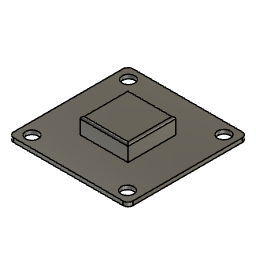
GYSFDMAXB (Autodesk Fusion 360 design; units mm, degrees)
Autodesk Fusion 360 part; units mm, degrees
sketch "スケッチ1" plane through (0, 0, 0) normal (0, 0, 1) x (1, 0, 0)
  line L0 (0, 0) -> (30, 0)
  line L1 (30, 0) -> (0, 0)
  line L2 (0, 0) -> (0, 30)
  line L3 (0, 30) -> (30, 30)
  line L4 (30, 30) -> (30, 0)
  line L5 (0, 0) -> (1.25, 0)
  line L6 (0, 0) -> (0, 1.25)
  arc A0 (0, 1.25) -> (1.25, 0) centre (1.25, 1.25) ccw
  arc A1 (1.25, 30) -> (0, 28.75) centre (1.25, 28.75) ccw
  arc A2 (30, 28.75) -> (28.75, 30) centre (28.75, 28.75) ccw
  arc A3 (28.75, 0) -> (30, 1.25) centre (28.75, 1.25) ccw
  line L7 (0, 30) -> (0, 28.73)
  circle A4 centre (3, 27.13) radius 1.6
  circle A5 centre (27, 27.13) radius 1.6
  circle A6 centre (27, 2.87) radius 1.6
  circle A7 centre (3, 2.87) radius 1.6
  dimension "d1" = 30
  dimension "d2" = 1.25
  dimension "d3" = 1.25
  dimension "d4" = 1.27
  dimension "d6" = 3.2
  constraint coincident L0.start L1.end
  constraint horizontal L0
  constraint horizontal L1
  constraint vertical L2
  constraint horizontal L3
  constraint vertical L4
  constraint perpendicular L2 L5
  constraint perpendicular L5 L6
  constraint perpendicular L3 L7
  measures "d1" distance of L0.start L0.end
  measures "d2" distance of L0.start L5.end
  measures "d3" distance of L0.start L6.end
  measures "d4" distance of L2.end L7.end
  measures "d6" diameter of A4
extrude "押し出し1" add sketch "スケッチ1" along normal blind 1 contours L0 L1 L2 L3 L4 A0 A1 A2 A3 L7
sketch "スケッチ2" plane through (0, 0, 1) normal (0, 0, 1) x (-1, 0, 0)
  circle A0 centre (-3, -27.13) radius 1.6
  circle A1 centre (-3, -2.87) radius 1.6
  circle A2 centre (-27, -2.87) radius 1.6
  circle A3 centre (-27, -27.13) radius 1.6
  arc A4 (-30, -28.75) -> (-28.75, -30) centre (-28.75, -28.75) ccw
  line L0 (-28.75, -30) -> (-1.25, -30)
  arc A5 (-1.25, -30) -> (0, -28.75) centre (-1.25, -28.75) ccw
  line L1 (0, -28.75) -> (0, -1.25)
  arc A6 (0, -1.25) -> (-1.25, 0) centre (-1.25, -1.25) ccw
  line L2 (-1.25, 0) -> (-28.75, 0)
  arc A7 (-28.75, 0) -> (-30, -1.25) centre (-28.75, -1.25) ccw
  line L3 (-30, -1.25) -> (-30, -28.75)
  line L4 (-8, -22) -> (-8, -8)
  line L5 (-8, -8) -> (-22, -8)
  line L6 (-22, -8) -> (-22, -22)
  line L7 (-22, -22) -> (-8, -22)
  constraint vertical L4
  constraint perpendicular L4 L5
  constraint perpendicular L5 L6
  constraint perpendicular L4 L7
sketch "スケッチ3" plane through (0, 0, 1) normal (0, 0, 1) x (-1, 0, 0)
  circle A0 centre (-3, -27.13) radius 1.6
  circle A1 centre (-3, -2.87) radius 1.6
  circle A2 centre (-27, -2.87) radius 1.6
  circle A3 centre (-27, -27.13) radius 1.6
  arc A4 (-30, -28.75) -> (-28.75, -30) centre (-28.75, -28.75) ccw
  line L0 (-28.75, -30) -> (-1.25, -30)
  arc A5 (-1.25, -30) -> (0, -28.75) centre (-1.25, -28.75) ccw
  line L1 (0, -28.75) -> (0, -1.25)
  arc A6 (0, -1.25) -> (-1.25, 0) centre (-1.25, -1.25) ccw
  line L2 (-1.25, 0) -> (-28.75, 0)
  arc A7 (-28.75, 0) -> (-30, -1.25) centre (-28.75, -1.25) ccw
  line L3 (-30, -1.25) -> (-30, -28.75)
  line L4 (-9, -21) -> (-9, -9)
  line L5 (-9, -9) -> (-21, -9)
  line L6 (-21, -9) -> (-21, -21)
  line L7 (-21, -21) -> (-9, -21)
  constraint vertical L4
  constraint perpendicular L4 L5
  constraint perpendicular L5 L6
  constraint perpendicular L4 L7
extrude "押し出し3" add sketch "スケッチ3" along normal blind 4 contours L4 L5 L6 L7
fillet "フィレット2" radius 0.5 1 faces at (13, 17, 5)
extrude "押し出し2" [suppressed]
fillet "フィレット1" [suppressed]
